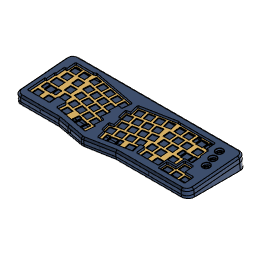
Trifecta (Autodesk Fusion 360 design; units mm, degrees)
Autodesk Fusion 360 part; units mm, degrees
(part 1 of 4)
sketch "plate" plane through (0, 0, 0) normal (0, 0, 1) x (1, 0, 0)
  arc A0 (312.6199, 117.774) -> (314.8699, 115.524) centre (314.8699, 117.774) ccw
  arc A1 (43.5915, -1.55) -> (40.3415, 1.7) centre (43.5915, 1.7) cw
  arc A2 (36.6259, 37.3436) -> (37.6259, 38.3436) centre (36.6259, 38.3436) ccw
  line L0 (175.886, -4.2231) -> (175.7904, -3.6814)
  arc A3 (112.7826, -2.4653) -> (110.9577, 0.1414) centre (110.5668, -2.0744) ccw
  arc A4 (31.0509, 50.8429) -> (30.0509, 49.8429) centre (31.0509, 49.8429) ccw
  arc A5 (179.6512, -6.859) -> (175.886, -4.2231) centre (179.0866, -3.6585) cw
  arc A6 (86.8114, 4.4012) -> (85.6822, 4.5) centre (85.6822, -2) ccw
  line L1 (47.3415, 2.25) -> (47.3415, 1.7)
  line L2 (-3.4991, 10) -> (-3.4991, 110.024)
  line L3 (312.6199, 118.324) -> (312.6199, 117.774)
  line L4 (26.1441, 107.024) -> (12.1447, 107.024)
  arc A7 (47.3415, 1.7) -> (44.0915, -1.55) centre (44.0915, 1.7) cw
  arc A8 (182.7796, -3.007) -> (180.1436, -6.7722) centre (179.579, -3.5716) cw
  line L5 (308.8699, 121.574) -> (309.3699, 121.574)
  line L6 (110.9577, 0.1414) -> (86.8114, 4.4012)
  line L7 (284.8904, 2.25) -> (284.8904, 1.7)
  line L8 (30.0509, 49.8429) -> (30.0509, 38.3436)
  arc A9 (115.323, -6.7722) -> (112.687, -3.007) centre (115.8876, -3.5716) cw
  line L9 (45.194, 107.024) -> (31.1947, 107.024)
  line L10 (112.687, -3.007) -> (112.7826, -2.4653)
  line L11 (352.994, 4.5) -> (287.1404, 4.5)
  circle A10 centre (133.6233, 118.074) radius 1.55
  arc A11 (277.8904, 2.25) -> (275.6404, 4.5) centre (275.6404, 2.25) ccw
  line L12 (12.0004, 37.3436) -> (6.4253, 37.3436)
  line L13 (40.3415, 1.7) -> (40.3415, 2.25)
  line L14 (305.6199, 117.774) -> (305.6199, 118.324)
  arc A12 (358.494, 10) -> (352.994, 4.5) centre (352.994, 10) cw
  line L15 (12.1447, 93.0243) -> (26.1441, 93.0243)
  line L16 (259.795, 93.0243) -> (273.794, 93.0243)
  line L17 (36.6259, 50.8429) -> (31.0509, 50.8429)
  line L18 (173.1838, -1.8565) -> (149.035, -6.1164)
  line L19 (146.4291, -6.1164) -> (122.2828, -1.8566)
  line L20 (180.1436, -6.7722) -> (179.6512, -6.859)
  line L21 (240.745, 107.024) -> (240.745, 93.0243)
  line L22 (208.6577, 4.4012) -> (184.5089, 0.1413)
  arc A13 (122.2828, -1.8566) -> (119.6762, -3.6815) centre (121.8919, -4.0724) ccw
  arc A14 (184.5089, 0.1413) -> (182.684, -2.4654) centre (184.8998, -2.0745) ccw
  arc A15 (40.3415, 2.25) -> (38.0915, 4.5) centre (38.0915, 2.25) ccw
  arc A16 (49.5915, 4.5) -> (47.3415, 2.25) centre (49.5915, 2.25) ccw
  line L23 (38.0915, 4.5) -> (2.0009, 4.5)
  arc A17 (13.0004, 38.3436) -> (12.0004, 37.3436) centre (12.0004, 38.3436) cw
  line L24 (115.8154, -6.859) -> (115.323, -6.7722)
  line L25 (288.37, 93.0243) -> (288.37, 107.024)
  arc A18 (309.3699, 121.574) -> (312.6199, 118.324) centre (309.3699, 118.324) cw
  line L26 (119.6762, -3.6815) -> (119.5806, -4.2231)
  line L27 (277.8904, 1.7) -> (277.8904, 2.25)
  arc A19 (303.3699, 115.524) -> (305.6199, 117.774) centre (303.3699, 117.774) ccw
  line L28 (358.494, 110.024) -> (358.494, 10)
  line L29 (31.0509, 37.3436) -> (36.6259, 37.3436)
  line L30 (13.0004, 49.8429) -> (13.0004, 38.3436)
  line L31 (182.684, -2.4654) -> (182.7796, -3.007)
  line L32 (85.6822, 4.5) -> (49.5915, 4.5)
  line L33 (174.9478, 20.2574) -> (176.9451, 8.9317)
  line L34 (303.895, 106.9941) -> (303.895, 95.4943)
  line L35 (98.9566, 12.3811) -> (100.9548, 23.7064)
  line L36 (314.754, 69.8941) -> (309.18, 69.8941)
  line L37 (283.556, 57.3947) -> (283.556, 68.8941)
  arc A20 (106.4177, 11.0651) -> (105.2592, 10.254) centre (105.4329, 11.2388) cw
  arc A21 (284.8904, 1.7) -> (281.6404, -1.55) centre (281.6404, 1.7) cw
  line L38 (304.895, 94.4943) -> (310.47, 94.4943)
  arc A22 (303.895, 95.4943) -> (304.895, 94.4943) centre (304.895, 95.4943) ccw
  line L39 (105.2592, 10.254) -> (99.7677, 11.2225)
  arc A23 (286.844, 95.4943) -> (285.844, 94.4943) centre (285.844, 95.4943) cw
  line L40 (279.269, 95.4943) -> (279.269, 106.9941)
  line L41 (315.754, 57.3947) -> (315.754, 68.8941)
  line L42 (130.6683, 6.7899) -> (132.6638, 18.1157)
  arc A24 (2.0009, 4.5) -> (-3.4991, 10) centre (2.0009, 10) cw
  arc A25 (287.1404, 4.5) -> (284.8904, 2.25) centre (287.1404, 2.25) ccw
  arc A26 (5.4253, 49.8429) -> (6.4253, 50.8429) centre (6.4253, 49.8429) cw
  line L43 (286.844, 106.9941) -> (286.844, 95.4943)
  arc A27 (314.754, 56.3947) -> (315.754, 57.3947) centre (314.754, 57.3947) ccw
  arc A28 (285.844, 107.9941) -> (286.844, 106.9941) centre (285.844, 106.9941) cw
  arc A29 (209.7869, 4.5) -> (208.6577, 4.4012) centre (209.7869, -2) ccw
  arc A30 (309.18, 69.8941) -> (308.18, 68.8941) centre (309.18, 68.8941) ccw
  line L44 (37.6259, 38.3436) -> (37.6259, 49.8429)
  arc A31 (305.6199, 118.324) -> (308.8699, 121.574) centre (308.8699, 118.324) cw
  arc A32 (126.3618, 20.2415) -> (125.2035, 19.4302) centre (126.1883, 19.2566) ccw
  arc A33 (191.7396, 23.2186) -> (192.5507, 24.3771) centre (192.7244, 23.3923) cw
  line L45 (281.6404, -1.55) -> (281.1404, -1.55)
  arc A34 (290.13, 69.8941) -> (291.13, 68.8941) centre (290.13, 68.8941) cw
  arc A35 (281.1404, -1.55) -> (277.8904, 1.7) centre (281.1404, 1.7) cw
  line L46 (227.1216, 115.524) -> (303.3699, 115.524)
  line L47 (124.0183, 6.9465) -> (129.5099, 5.9786)
  line L48 (131.8525, 19.274) -> (126.3618, 20.2415)
  line L49 (44.0915, -1.55) -> (43.5915, -1.55)
  arc A36 (30.0509, 38.3436) -> (31.0509, 37.3436) centre (31.0509, 38.3436) ccw
  line L50 (291.13, 68.8941) -> (291.13, 57.3947)
  arc A37 (310.47, 94.4943) -> (311.47, 95.4943) centre (310.47, 95.4943) ccw
  line L51 (309.18, 56.3947) -> (314.754, 56.3947)
  arc A38 (149.035, -6.1164) -> (146.4291, -6.1164) centre (147.7321, 1.2696) cw
  line L52 (275.6404, 4.5) -> (209.7869, 4.5)
  line L53 (125.2035, 19.4302) -> (123.207, 8.1049)
  line L54 (192.5507, 24.3771) -> (198.0375, 25.3445)
  arc A39 (119.5806, -4.2231) -> (115.8154, -6.859) centre (116.38, -3.6585) cw
  arc A40 (107.6038, 23.5487) -> (108.4148, 22.3903) centre (107.43, 22.564) cw
  line L55 (314.8699, 115.524) -> (352.994, 115.524)
  arc A41 (170.6459, 6.8059) -> (169.4875, 7.6172) centre (170.4724, 7.7907) cw
  arc A42 (167.4915, 18.9424) -> (168.3027, 20.1008) centre (168.4764, 19.116) cw
  arc A43 (99.7677, 11.2225) -> (98.9566, 12.3811) centre (99.9414, 12.2073) cw
  arc A44 (6.4253, 37.3436) -> (5.4253, 38.3436) centre (6.4253, 38.3436) cw
  arc A45 (291.13, 57.3947) -> (290.13, 56.3947) centre (290.13, 57.3947) cw
  line L56 (102.1133, 24.5174) -> (107.6038, 23.5487)
  arc A46 (175.7904, -3.6814) -> (173.1838, -1.8565) centre (173.5747, -4.0723) ccw
  arc A47 (352.994, 115.524) -> (358.494, 110.024) centre (352.994, 110.024) cw
  arc A48 (37.6259, 49.8429) -> (36.6259, 50.8429) centre (36.6259, 49.8429) ccw
  arc A49 (311.47, 106.9941) -> (310.47, 107.9941) centre (310.47, 106.9941) ccw
  line L57 (310.47, 107.9941) -> (304.895, 107.9941)
  line L58 (108.4148, 22.3903) -> (106.4177, 11.0651)
  line L59 (5.4253, 38.3436) -> (5.4253, 49.8429)
  arc A50 (129.5099, 5.9786) -> (130.6683, 6.7899) centre (129.6834, 6.9634) ccw
  arc A51 (100.9548, 23.7064) -> (102.1133, 24.5174) centre (101.9395, 23.5327) cw
  arc A52 (308.18, 57.3947) -> (309.18, 56.3947) centre (309.18, 57.3947) ccw
  line L60 (284.556, 69.8941) -> (290.13, 69.8941)
  line L61 (308.18, 68.8941) -> (308.18, 57.3947)
  line L62 (6.4253, 50.8429) -> (12.0004, 50.8429)
  arc A53 (315.754, 68.8941) -> (314.754, 69.8941) centre (314.754, 68.8941) ccw
  line L63 (290.13, 56.3947) -> (284.556, 56.3947)
  arc A54 (201.1942, 13.2086) -> (200.3832, 12.0501) centre (200.2094, 13.0348) cw
  arc A55 (173.7893, 21.0686) -> (174.9478, 20.2574) centre (173.963, 20.0838) cw
  line L64 (169.4875, 7.6172) -> (167.4915, 18.9424)
  arc A56 (123.207, 8.1049) -> (124.0183, 6.9465) centre (124.1918, 7.9313) ccw
  arc A57 (198.0375, 25.3445) -> (199.1959, 24.5335) centre (198.2111, 24.3597) cw
  line L65 (280.269, 107.9941) -> (285.844, 107.9941)
  arc A58 (304.895, 107.9941) -> (303.895, 106.9941) centre (304.895, 106.9941) ccw
  line L66 (200.3832, 12.0501) -> (194.8954, 11.0818)
  line L67 (285.844, 94.4943) -> (280.269, 94.4943)
  arc A59 (132.6638, 18.1157) -> (131.8525, 19.274) centre (131.679, 18.2892) ccw
  arc A60 (284.556, 56.3947) -> (283.556, 57.3947) centre (284.556, 57.3947) cw
  arc A61 (279.269, 106.9941) -> (280.269, 107.9941) centre (280.269, 106.9941) cw
  arc A62 (283.556, 68.8941) -> (284.556, 69.8941) centre (284.556, 68.8941) cw
  line L68 (168.3027, 20.1008) -> (173.7893, 21.0686)
  arc A63 (12.0004, 50.8429) -> (13.0004, 49.8429) centre (12.0004, 49.8429) cw
  line L69 (193.7369, 11.8929) -> (191.7396, 23.2186)
  arc A64 (176.9451, 8.9317) -> (176.1339, 7.7732) centre (175.9603, 8.758) cw
  arc A65 (280.269, 94.4943) -> (279.269, 95.4943) centre (280.269, 95.4943) cw
  arc A66 (194.8954, 11.0818) -> (193.7369, 11.8929) centre (194.7217, 12.0666) cw
  line L70 (311.47, 95.4943) -> (311.47, 106.9941)
  line L71 (176.1339, 7.7732) -> (170.6459, 6.8059)
  line L72 (199.1959, 24.5335) -> (201.1942, 13.2086)
  line L73 (209.276, 26.3412) -> (223.063, 28.7721)
  line L74 (307.132, 26.0615) -> (293.132, 26.0615)
  line L75 (117.549, 25.9388) -> (103.762, 28.3697)
  line L76 (101.221, 43.0332) -> (98.7887, 29.2475)
  line L77 (352.994, 115.024) -> (314.8699, 115.024)
  line L78 (215.434, 32.5548) -> (213.003, 46.3419)
  line L79 (229.222, 34.9856) -> (215.434, 32.5548)
  line L80 (307.132, 12.062) -> (307.132, 26.0615)
  line L81 (5.0009, 16.8245) -> (19.0004, 16.8245)
  line L82 (196.674, 29.2475) -> (194.243, 43.0332)
  line L83 (87.4339, 45.4642) -> (101.221, 43.0332)
  line L84 (312.182, 12.062) -> (326.182, 12.062)
  line L85 (293.132, 26.0615) -> (293.132, 12.062)
  line L86 (293.132, 12.062) -> (307.132, 12.062)
  line L87 (210.461, 31.6784) -> (196.674, 29.2475)
  line L88 (28.812, 16.8245) -> (42.8128, 16.8245)
  line L89 (226.791, 48.7729) -> (229.222, 34.9856)
  line L90 (66.2411, 34.9856) -> (68.6731, 48.7729)
  line L91 (106.193, 42.1569) -> (119.98, 39.726)
  line L92 (312.182, 45.1115) -> (312.182, 31.112)
  line L93 (124.955, 38.8482) -> (138.741, 36.4173)
  line L94 (326.182, 12.062) -> (326.182, 26.0615)
  line L95 (208.03, 45.4642) -> (210.461, 31.6784)
  line L96 (86.1882, 26.3412) -> (83.7558, 12.5525)
  arc A67 (357.994, 110.024) -> (352.994, 115.024) centre (352.994, 110.024) ccw
  line L97 (213.003, 46.3419) -> (226.791, 48.7729)
  line L98 (194.243, 43.0332) -> (208.03, 45.4642)
  line L99 (42.8128, 16.8245) -> (42.8128, 30.824)
  line L100 (309.3699, 121.074) -> (308.8699, 121.074)
  line L101 (19.0004, 16.8245) -> (19.0004, 30.824)
  line L102 (69.9685, 14.9848) -> (72.3995, 28.7721)
  line L103 (138.741, 36.4173) -> (136.31, 22.6315)
  line L104 (103.762, 28.3697) -> (106.193, 42.1569)
  line L105 (331.232, 26.0615) -> (331.232, 12.062)
  line L106 (223.063, 28.7721) -> (225.494, 14.9848)
  line L107 (156.722, 36.4173) -> (170.509, 38.8482)
  line L108 (72.3995, 28.7721) -> (86.1882, 26.3412)
  arc A68 (306.1199, 117.774) -> (303.3699, 115.024) centre (303.3699, 117.774) cw
  arc A69 (42.875, 117.774) -> (40.125, 115.024) centre (40.125, 117.774) cw
  line L109 (357.994, 10) -> (357.994, 110.024)
  line L110 (46.8415, 1.7) -> (46.8415, 2.25)
  line L111 (326.182, 45.1115) -> (312.182, 45.1115)
  line L112 (176.2828, -3.5946) -> (176.3784, -4.1362)
  line L113 (42.8128, 30.824) -> (28.812, 30.824)
  line L114 (306.1199, 118.324) -> (306.1199, 117.774)
  line L115 (184.4221, 0.6337) -> (208.5708, 4.8936)
  arc A70 (139.3733, 115.024) -> (136.6233, 117.774) centre (139.3733, 117.774) cw
  line L116 (82.459, 46.3419) -> (80.0283, 32.5548)
  line L117 (83.7558, 12.5525) -> (69.9685, 14.9848)
  line L118 (326.182, 26.0615) -> (312.182, 26.0615)
  line L119 (159.153, 22.6315) -> (156.722, 36.4173)
  line L120 (175.482, 39.726) -> (189.27, 42.1569)
  line L121 (19.0004, 30.824) -> (5.0009, 30.824)
  line L122 (345.232, 12.062) -> (345.232, 26.0615)
  line L123 (331.232, 12.062) -> (345.232, 12.062)
  line L124 (98.7887, 29.2475) -> (85.0015, 31.6784)
  line L125 (326.182, 31.112) -> (326.182, 45.1115)
  line L126 (218.3716, 118.324) -> (218.3716, 117.774)
  line L127 (136.31, 22.6315) -> (122.524, 25.0624)
  line L128 (136.6233, 117.774) -> (136.6233, 118.324)
  line L129 (68.6731, 48.7729) -> (82.459, 46.3419)
  line L130 (225.494, 14.9848) -> (211.708, 12.5525)
  line L131 (80.0283, 32.5548) -> (66.2411, 34.9856)
  line L132 (5.0009, 30.824) -> (5.0009, 16.8245)
  arc A71 (312.1199, 118.324) -> (309.3699, 121.074) centre (309.3699, 118.324) ccw
  line L133 (2.0009, 5) -> (38.0915, 5)
  line L134 (345.232, 26.0615) -> (331.232, 26.0615)
  line L135 (211.708, 12.5525) -> (209.276, 26.3412)
  line L136 (170.509, 38.8482) -> (172.94, 25.0624)
  line L137 (191.7, 28.3697) -> (177.913, 25.9388)
  arc A72 (314.8699, 115.024) -> (312.1199, 117.774) centre (314.8699, 117.774) cw
  line L138 (172.94, 25.0624) -> (159.153, 22.6315)
  line L139 (177.913, 25.9388) -> (175.482, 39.726)
  line L140 (189.27, 42.1569) -> (191.7, 28.3697)
  line L141 (312.182, 26.0615) -> (312.182, 12.062)
  line L142 (312.182, 31.112) -> (326.182, 31.112)
  line L143 (28.812, 30.824) -> (28.812, 16.8245)
  line L144 (85.0015, 31.6784) -> (87.4339, 45.4642)
  line L145 (113.275, -2.5522) -> (113.1794, -3.0938)
  line L146 (312.1199, 117.774) -> (312.1199, 118.324)
  line L147 (122.524, 25.0624) -> (124.955, 38.8482)
  line L148 (119.98, 39.726) -> (117.549, 25.9388)
  arc A73 (46.8415, 2.25) -> (49.5915, 5) centre (49.5915, 2.25) cw
  line L149 (42.875, 118.324) -> (42.875, 117.774)
  arc A74 (44.0915, -1.05) -> (46.8415, 1.7) centre (44.0915, 1.7) ccw
  arc A75 (2.0009, 115.024) -> (-2.9991, 110.024) centre (2.0009, 110.024) ccw
  arc A76 (218.3716, 117.774) -> (215.6216, 115.024) centre (215.6216, 117.774) cw
  line L150 (221.6216, 121.074) -> (221.1216, 121.074)
  arc A77 (308.8699, 121.074) -> (306.1199, 118.324) centre (308.8699, 118.324) ccw
  arc A78 (133.3733, 121.074) -> (130.6233, 118.324) centre (133.3733, 118.324) ccw
  arc A79 (119.1838, -3.5946) -> (122.3697, -1.3642) centre (121.8919, -4.0724) cw
  line L151 (115.4099, -6.2798) -> (115.9023, -6.3666)
  line L152 (224.3716, 117.774) -> (224.3716, 118.324)
  arc A80 (113.1794, -3.0938) -> (115.4099, -6.2798) centre (115.8876, -3.5716) ccw
  arc A81 (-2.9991, 10) -> (2.0009, 5) centre (2.0009, 10) ccw
  line L153 (49.5915, 5) -> (85.6822, 5)
  line L154 (119.0882, -4.1362) -> (119.1838, -3.5946)
  arc A82 (38.0915, 5) -> (40.8415, 2.25) centre (38.0915, 2.25) cw
  line L155 (303.3699, 115.024) -> (227.1216, 115.024)
  line L156 (48.875, 117.774) -> (48.875, 118.324)
  arc A83 (173.0969, -1.3641) -> (176.2828, -3.5946) centre (173.5747, -4.0723) cw
  line L157 (182.2872, -3.0939) -> (182.1916, -2.5522)
  line L158 (45.4822, 49.874) -> (45.4822, 35.8743)
  line L159 (195.341, 62.5711) -> (197.772, 48.7839)
  arc A84 (146.516, -5.624) -> (148.9482, -5.624) centre (147.7321, 1.2696) ccw
  line L160 (127.8733, 115.024) -> (51.625, 115.024)
  line L161 (122.3697, -1.3642) -> (146.516, -5.624)
  arc A85 (51.625, 115.024) -> (48.875, 117.774) centre (51.625, 117.774) cw
  arc A86 (85.6822, 5) -> (86.8983, 4.8935) centre (85.6822, -2) cw
  line L162 (133.8733, 121.074) -> (133.3733, 121.074)
  line L163 (281.1404, -1.05) -> (281.6404, -1.05)
  line L164 (349.994, 68.924) -> (335.995, 68.924)
  line L165 (281.226, 49.874) -> (281.226, 35.8743)
  arc A87 (208.5708, 4.8936) -> (209.7869, 5) centre (209.7869, -2) cw
  arc A88 (45.625, 121.074) -> (42.875, 118.324) centre (45.625, 118.324) ccw
  arc A89 (176.3784, -4.1362) -> (179.5643, -6.3666) centre (179.0866, -3.6585) ccw
  arc A90 (275.6404, 5) -> (278.3904, 2.25) centre (275.6404, 2.25) cw
  line L166 (215.6216, 115.024) -> (139.3733, 115.024)
  arc A91 (111.0446, 0.6338) -> (113.275, -2.5522) centre (110.5668, -2.0744) cw
  arc A92 (227.1216, 115.024) -> (224.3716, 117.774) centre (227.1216, 117.774) cw
  line L167 (40.125, 115.024) -> (2.0009, 115.024)
  line L168 (179.5643, -6.3666) -> (180.0567, -6.2798)
  line L169 (278.3904, 2.25) -> (278.3904, 1.7)
  arc A93 (48.875, 118.324) -> (46.125, 121.074) centre (46.125, 118.324) ccw
  line L170 (-2.9991, 110.024) -> (-2.9991, 10)
  line L171 (295.225, 35.8743) -> (295.225, 49.874)
  arc A94 (130.6233, 117.774) -> (127.8733, 115.024) centre (127.8733, 117.774) cw
  line L172 (235.982, 49.874) -> (235.982, 35.8743)
  line L173 (209.7869, 5) -> (275.6404, 5)
  arc A95 (352.994, 5) -> (357.994, 10) centre (352.994, 10) ccw
  arc A96 (221.1216, 121.074) -> (218.3716, 118.324) centre (221.1216, 118.324) ccw
  line L174 (116.451, 45.4752) -> (118.882, 59.2624)
  line L175 (46.125, 121.074) -> (45.625, 121.074)
  arc A97 (40.8415, 1.7) -> (43.5915, -1.05) centre (43.5915, 1.7) ccw
  line L176 (130.6233, 118.324) -> (130.6233, 117.774)
  arc A98 (136.6233, 118.324) -> (133.8733, 121.074) centre (133.8733, 118.324) ccw
  line L177 (249.982, 49.874) -> (235.982, 49.874)
  line L178 (86.8983, 4.8935) -> (111.0446, 0.6338)
  line L179 (45.4822, 35.8743) -> (59.4815, 35.8743)
  line L180 (14.5259, 49.874) -> (28.5254, 49.874)
  arc A99 (180.0567, -6.2798) -> (182.2872, -3.0939) centre (179.579, -3.5716) ccw
  line L181 (255.032, 49.874) -> (255.032, 35.8743)
  line L182 (28.5254, 35.8743) -> (14.5259, 35.8743)
  line L183 (43.5915, -1.05) -> (44.0915, -1.05)
  line L184 (165.224, 43.0445) -> (162.793, 56.8318)
  arc A100 (182.1916, -2.5522) -> (184.4221, 0.6337) centre (184.8998, -2.0745) cw
  line L185 (106.805, 13.2623) -> (106.8051, 13.2623)
  line L186 (269.032, 35.8743) -> (269.032, 49.874)
  line L187 (132.669, 56.8318) -> (130.238, 43.0445)
  line L188 (148.9482, -5.624) -> (173.0969, -1.3641)
  arc A101 (115.9023, -6.3666) -> (119.0882, -4.1362) centre (116.38, -3.6585) ccw
  arc A102 (224.3716, 118.324) -> (221.6216, 121.074) centre (221.6216, 118.324) ccw
  line L189 (197.772, 48.7839) -> (183.986, 46.3532)
  line L190 (176.444, 20.5521) -> (190.233, 22.9829)
  line L191 (235.982, 35.8743) -> (249.982, 35.8743)
  line L192 (335.995, 54.9243) -> (349.994, 54.9243)
  line L193 (281.226, 35.8743) -> (295.225, 35.8743)
  line L194 (249.982, 35.8743) -> (249.982, 49.874)
  line L195 (107.49, 8.3688) -> (109.921, 22.1561)
  line L196 (28.5254, 49.874) -> (28.5254, 35.8743)
  line L197 (40.8415, 2.25) -> (40.8415, 1.7)
  arc A103 (284.3904, 2.25) -> (287.1404, 5) centre (287.1404, 2.25) cw
  line L198 (280.938, 16.8245) -> (280.938, 30.824)
  line L199 (266.937, 30.824) -> (266.937, 16.8245)
  line L200 (81.3608, 65.8784) -> (95.148, 63.4478)
  line L201 (181.555, 60.1405) -> (195.341, 62.5711)
  line L202 (52.8147, 54.9243) -> (52.8147, 68.924)
  line L203 (111.478, 46.3532) -> (97.6905, 48.7839)
  line L204 (211.077, 84.6899) -> (224.864, 87.1209)
  line L205 (269.032, 73.9743) -> (269.032, 87.974)
  line L206 (306.655, 54.9243) -> (292.655, 54.9243)
  line L207 (59.4815, 35.8743) -> (59.4815, 49.874)
  line L208 (189.775, 66.7177) -> (175.988, 64.2867)
  line L209 (345.232, 87.974) -> (331.232, 87.974)
  line L210 (176.582, 59.2624) -> (179.013, 45.4752)
  line L211 (221.506, 52.9689) -> (219.075, 66.7561)
  line L212 (284.3904, 1.7) -> (284.3904, 2.25)
  line L213 (255.032, 35.8743) -> (269.032, 35.8743)
  line L214 (118.882, 59.2624) -> (132.669, 56.8318)
  line L215 (227.295, 73.3337) -> (213.509, 70.9027)
  line L216 (113.909, 60.1405) -> (111.478, 46.3532)
  line L217 (269.032, 87.974) -> (255.032, 87.974)
  line L218 (52.8147, 68.924) -> (38.8137, 68.924)
  line L219 (14.5259, 35.8743) -> (14.5259, 49.874)
  line L220 (257.125, 16.8245) -> (257.125, 30.824)
  arc A104 (281.6404, -1.05) -> (284.3904, 1.7) centre (281.6404, 1.7) ccw
  line L221 (269.032, 49.874) -> (255.032, 49.874)
  line L222 (109.921, 22.1561) -> (123.708, 19.7253)
  line L223 (178.876, 6.7634) -> (176.444, 20.5521)
  line L224 (280.938, 30.824) -> (266.937, 30.824)
  line L225 (121.277, 5.9366) -> (107.49, 8.3688)
  line L226 (130.238, 43.0445) -> (116.451, 45.4752)
  line L227 (266.937, 16.8245) -> (280.938, 16.8245)
  line L228 (162.793, 56.8318) -> (176.582, 59.2624)
  line L229 (107.6039, 17.7917) -> (107.603, 17.7919)
  line L230 (59.4815, 49.874) -> (45.4822, 49.874)
  line L231 (335.995, 68.924) -> (335.995, 54.9243)
  line L232 (192.664, 9.1957) -> (178.876, 6.7634)
  line L233 (168.785, 11.5852) -> (168.7882, 11.5858)
  line L234 (183.986, 46.3532) -> (181.555, 60.1405)
  line L235 (235.293, 55.3999) -> (221.506, 52.9689)
  line L236 (60.1694, 55.3999) -> (62.6001, 69.1871)
  line L237 (219.075, 66.7561) -> (232.862, 69.1871)
  line L238 (179.013, 45.4752) -> (165.224, 43.0445)
  line L239 (295.225, 49.874) -> (281.226, 49.874)
  line L240 (187.343, 80.5049) -> (189.775, 66.7177)
  line L241 (349.994, 54.9243) -> (349.994, 68.924)
  line L242 (345.232, 73.9743) -> (345.232, 87.974)
  line L243 (177.334, 6.7262) -> (177.334, 6.7262)
  line L244 (173.557, 78.0743) -> (187.343, 80.5049)
  line L245 (190.233, 22.9829) -> (192.664, 9.1956)
  line L246 (168.582, 77.1962) -> (171.013, 63.4104)
  line L247 (255.032, 73.9743) -> (269.032, 73.9743)
  line L248 (38.8137, 54.9243) -> (52.8147, 54.9243)
  line L249 (243.126, 30.824) -> (243.126, 16.8245)
  line L250 (257.125, 30.824) -> (243.126, 30.824)
  arc A105 (278.3904, 1.7) -> (281.1404, -1.05) centre (281.1404, 1.7) ccw
  line L251 (287.1404, 5) -> (352.994, 5)
  line L252 (123.708, 19.7253) -> (121.277, 5.9366)
  line L253 (95.148, 63.4478) -> (92.7171, 49.6605)
  line L254 (175.988, 64.2867) -> (173.557, 78.0743)
  line L255 (58.7872, 74.9886) -> (61.2179, 88.7748)
  line L256 (213.509, 70.9027) -> (211.077, 84.6899)
  line L257 (76.3873, 66.7561) -> (73.9567, 52.9689)
  line L258 (243.126, 16.8245) -> (257.125, 16.8245)
  line L259 (110.096, 65.9405) -> (96.3083, 68.3715)
  line L260 (275.7, 68.924) -> (261.699, 68.924)
  line L261 (171.013, 63.4104) -> (157.226, 60.9783)
  line L262 (75.0051, 86.3438) -> (72.5745, 72.5565)
  line L263 (292.655, 68.924) -> (306.655, 68.924)
  line L264 (249.982, 73.9743) -> (249.982, 87.974)
  line L265 (311.894, 87.974) -> (297.895, 87.974)
  line L266 (61.2179, 88.7748) -> (75.0051, 86.3438)
  line L267 (100.122, 62.5711) -> (113.909, 60.1405)
  line L268 (77.5476, 71.6802) -> (79.9786, 85.4675)
  line L269 (179.629, 98.4885) -> (193.416, 100.919)
  line L270 (182.059, 84.7012) -> (179.629, 98.4885)
  line L271 (193.416, 100.919) -> (195.847, 87.1319)
  line L272 (12.6201, 54.9243) -> (26.6209, 54.9243)
  line L273 (224.864, 87.1209) -> (227.295, 73.3337)
  line L274 (255.032, 87.974) -> (255.032, 73.9743)
  line L275 (202.747, 49.6605) -> (200.314, 63.4478)
  line L276 (214.103, 65.8784) -> (216.534, 52.0912)
  line L277 (130.189, 95.9584) -> (143.976, 93.5274)
  line L278 (174.655, 97.6119) -> (177.086, 83.8232)
  line L279 (256.65, 68.924) -> (242.649, 68.924)
  line L280 (297.895, 87.974) -> (297.895, 73.9743)
  line L281 (242.649, 54.9243) -> (256.65, 54.9243)
  line L282 (97.6905, 48.7839) -> (100.122, 62.5711)
  line L283 (12.1447, 73.9743) -> (26.1441, 73.9743)
  line L284 (73.9567, 52.9689) -> (60.1694, 55.3999)
  line L285 (112.527, 79.7278) -> (110.096, 65.9405)
  line L286 (331.232, 87.974) -> (331.232, 73.9743)
  line L287 (35.9572, 87.974) -> (35.9572, 73.9743)
  line L288 (275.7, 54.9243) -> (275.7, 68.924)
  line L289 (235.982, 87.974) -> (235.982, 73.9743)
  line L290 (261.699, 68.924) -> (261.699, 54.9243)
  line L291 (38.8137, 68.924) -> (38.8137, 54.9243)
  line L292 (230.937, 107.535) -> (233.368, 93.7479)
  line L293 (111.428, 99.2657) -> (125.214, 96.8347)
  line L294 (160.868, 95.1812) -> (174.655, 97.6119)
  line L295 (79.9786, 85.4675) -> (93.7659, 83.0365)
  line L296 (232.862, 69.1871) -> (235.293, 55.3999)
  line L297 (200.314, 63.4478) -> (214.103, 65.8784)
  line L298 (331.232, 73.9743) -> (345.232, 73.9743)
  line L299 (306.655, 68.924) -> (306.655, 54.9243)
  line L300 (35.9572, 73.9743) -> (49.9565, 73.9743)
  line L301 (274.082, 87.974) -> (274.082, 73.9743)
  line L302 (256.65, 54.9243) -> (256.65, 68.924)
  line L303 (292.655, 54.9243) -> (292.655, 68.924)
  line L304 (62.6001, 69.1871) -> (76.3873, 66.7561)
  line L305 (154.795, 74.7656) -> (168.582, 77.1962)
  line L306 (216.534, 52.0912) -> (202.747, 49.6605)
  line L307 (117.5, 78.8515) -> (131.287, 76.4205)
  line L308 (78.9298, 52.0912) -> (81.3608, 65.8784)
  line L309 (208.536, 70.0264) -> (194.747, 67.5954)
  line L310 (311.894, 73.9743) -> (311.894, 87.974)
  line L311 (96.3083, 68.3715) -> (98.7393, 82.1588)
  line L312 (261.699, 54.9243) -> (275.7, 54.9243)
  line L313 (115.069, 65.0642) -> (117.5, 78.8515)
  line L314 (98.7393, 82.1588) -> (112.527, 79.7278)
  line L315 (26.6209, 54.9243) -> (26.6209, 68.924)
  line L316 (26.6209, 68.924) -> (12.6201, 68.924)
  line L317 (72.5745, 72.5565) -> (58.7872, 74.9886)
  line L318 (92.7171, 49.6605) -> (78.9298, 52.0912)
  line L319 (297.895, 73.9743) -> (311.894, 73.9743)
  line L320 (242.649, 68.924) -> (242.649, 54.9243)
  line L321 (157.226, 60.9783) -> (154.795, 74.7656)
  line L322 (106.455, 100.143) -> (104.024, 86.3547)
  line L323 (104.024, 86.3547) -> (90.2353, 88.7857)
  line L324 (49.9565, 87.974) -> (35.9572, 87.974)
  line L325 (194.747, 67.5954) -> (192.316, 81.3816)
  line L326 (288.082, 73.9743) -> (288.082, 87.974)
  line L327 (177.086, 83.8232) -> (163.299, 81.3925)
  line L328 (90.2353, 88.7857) -> (92.6663, 102.574)
  line L329 (206.105, 83.8122) -> (208.536, 70.0264)
  line L330 (26.1441, 87.974) -> (12.1447, 87.974)
  line L331 (93.7659, 83.0365) -> (91.3349, 69.2492)
  line L332 (108.996, 85.4784) -> (111.428, 99.2657)
  line L333 (214.607, 90.4392) -> (200.82, 88.0085)
  line L334 (233.368, 93.7479) -> (219.581, 91.3172)
  line L335 (212.176, 104.228) -> (214.607, 90.4392)
  line L336 (143.976, 93.5274) -> (141.544, 79.7387)
  line L337 (92.6663, 102.574) -> (106.455, 100.143)
  line L338 (219.581, 91.3172) -> (217.15, 105.104)
  line L339 (26.1441, 73.9743) -> (26.1441, 87.974)
  line L340 (274.082, 73.9743) -> (288.082, 73.9743)
  line L341 (217.15, 105.104) -> (230.937, 107.535)
  line L342 (127.758, 82.1697) -> (130.189, 95.9584)
  line L343 (288.082, 87.974) -> (274.082, 87.974)
  line L344 (12.1447, 87.974) -> (12.1447, 73.9743)
  line L345 (195.847, 87.1319) -> (182.059, 84.7012)
  line L346 (200.82, 88.0085) -> (198.389, 101.797)
  line L347 (49.9565, 73.9743) -> (49.9565, 87.974)
  line L348 (122.783, 83.0474) -> (108.996, 85.4784)
  line L349 (128.856, 62.6332) -> (115.069, 65.0642)
  line L350 (249.982, 87.974) -> (235.982, 87.974)
  line L351 (163.299, 81.3925) -> (160.868, 95.1812)
  line L352 (141.544, 79.7387) -> (127.758, 82.1697)
  line L353 (198.389, 101.797) -> (212.176, 104.228)
  line L354 (192.316, 81.3816) -> (206.105, 83.8122)
  line L355 (131.287, 76.4205) -> (128.856, 62.6332)
  line L356 (235.982, 73.9743) -> (249.982, 73.9743)
  line L357 (125.214, 96.8347) -> (122.783, 83.0474)
  line L358 (87.6928, 103.451) -> (85.2622, 89.6634)
  line L359 (12.6201, 68.924) -> (12.6201, 54.9243)
  arc A106 (137.1233, 117.774) -> (139.3733, 115.524) centre (139.3733, 117.774) ccw
  arc A107 (217.8716, 118.324) -> (221.1216, 121.574) centre (221.1216, 118.324) cw
  line L360 (71.476, 92.0944) -> (73.9069, 105.882)
  line L361 (326.47, 107.024) -> (326.47, 93.0243)
  line L362 (51.625, 115.524) -> (127.8733, 115.524)
  line L363 (26.1441, 93.0243) -> (26.1441, 107.024)
  arc A108 (133.8733, 121.574) -> (137.1233, 118.324) centre (133.8733, 118.324) cw
  line L364 (45.194, 93.0243) -> (45.194, 107.024)
  line L365 (259.795, 107.024) -> (259.795, 93.0243)
  line L366 (254.744, 107.024) -> (240.745, 107.024)
  arc A109 (-3.4991, 110.024) -> (2.0009, 115.524) centre (2.0009, 110.024) cw
  circle A110 centre (309.1199, 118.074) radius 1.55
  line L367 (254.744, 93.0243) -> (254.744, 107.024)
  line L368 (52.7142, 95.4017) -> (55.1448, 109.19)
  line L369 (31.1947, 93.0243) -> (45.194, 93.0243)
  line L370 (340.469, 93.0243) -> (340.469, 107.024)
  line L371 (45.625, 121.574) -> (46.125, 121.574)
  line L372 (139.3733, 115.524) -> (215.6216, 115.524)
  line L373 (240.745, 93.0243) -> (254.744, 93.0243)
  line L374 (12.1447, 107.024) -> (12.1447, 93.0243)
  line L375 (73.9069, 105.882) -> (87.6928, 103.451)
  line L376 (273.794, 93.0243) -> (273.794, 107.024)
  arc A111 (221.6216, 121.574) -> (224.8716, 118.324) centre (221.6216, 118.324) cw
  circle A112 centre (179.2893, -3.3688) radius 1.55
  circle A113 centre (116.1773, -3.3688) radius 1.55
  arc A114 (130.1233, 118.324) -> (133.3733, 121.574) centre (133.3733, 118.324) cw
  line L377 (91.3349, 69.2492) -> (77.5476, 71.6802)
  circle A115 centre (43.8415, 1.95) radius 1.55
  line L378 (49.375, 118.324) -> (49.375, 117.774)
  arc A116 (224.8716, 117.774) -> (227.1216, 115.524) centre (227.1216, 117.774) ccw
  line L379 (224.8716, 118.324) -> (224.8716, 117.774)
  line L380 (85.2622, 89.6634) -> (71.476, 92.0944)
  line L381 (137.1233, 118.324) -> (137.1233, 117.774)
  line L382 (55.1448, 109.19) -> (68.9335, 106.759)
  circle A117 centre (45.875, 118.074) radius 1.55
  circle A118 centre (281.3904, 1.95) radius 1.55
  line L383 (66.5014, 92.9707) -> (52.7142, 95.4017)
  line L384 (31.1947, 107.024) -> (31.1947, 93.0243)
  circle A119 centre (221.3716, 118.074) radius 1.55
  line L385 (288.37, 107.024) -> (302.369, 107.024)
  arc A120 (40.125, 115.524) -> (42.375, 117.774) centre (40.125, 117.774) ccw
  line L386 (2.0009, 115.524) -> (40.125, 115.524)
  line L387 (68.9335, 106.759) -> (66.5014, 92.9707)
  arc A121 (215.6216, 115.524) -> (217.8716, 117.774) centre (215.6216, 117.774) ccw
  arc A122 (46.125, 121.574) -> (49.375, 118.324) centre (46.125, 118.324) cw
  line L388 (326.47, 93.0243) -> (340.469, 93.0243)
  arc A123 (42.375, 118.324) -> (45.625, 121.574) centre (45.625, 118.324) cw
  arc A124 (127.8733, 115.524) -> (130.1233, 117.774) centre (127.8733, 117.774) ccw
  line L389 (133.3733, 121.574) -> (133.8733, 121.574)
  arc A125 (49.375, 117.774) -> (51.625, 115.524) centre (51.625, 117.774) ccw
  line L390 (221.1216, 121.574) -> (221.6216, 121.574)
  line L391 (273.794, 107.024) -> (259.795, 107.024)
  line L392 (217.8716, 117.774) -> (217.8716, 118.324)
  line L393 (130.1233, 117.774) -> (130.1233, 118.324)
  line L394 (340.469, 107.024) -> (326.47, 107.024)
  line L395 (302.369, 93.0243) -> (288.37, 93.0243)
  line L396 (302.369, 107.024) -> (302.369, 93.0243)
  line L397 (42.375, 117.774) -> (42.375, 118.324)
  line L398 (7.8576, 68.924) -> (7.8576, 54.9243)
  line L399 (7.8576, 68.924) -> (12.6201, 68.924)
  line L400 (7.8576, 54.9243) -> (12.6201, 54.9243)
  line L401 (359.744, 110.024) -> (359.744, 10)
  arc A126 (352.994, 3.25) -> (359.744, 10) centre (352.994, 10) ccw
  line L402 (352.994, 3.25) -> (287.1404, 3.25)
  arc A127 (287.1404, 3.25) -> (286.1404, 2.25) centre (287.1404, 2.25) ccw
  line L403 (286.1404, 2.25) -> (286.1404, 1.7)
  arc A128 (281.6404, -2.8) -> (286.1404, 1.7) centre (281.6404, 1.7) ccw
  line L404 (281.6404, -2.8) -> (281.1404, -2.8)
  arc A129 (276.6404, 1.7) -> (281.1404, -2.8) centre (281.1404, 1.7) ccw
  line L405 (276.6404, 1.7) -> (276.6404, 2.25)
  arc A130 (276.6404, 2.25) -> (275.6404, 3.25) centre (275.6404, 2.25) ccw
  line L406 (275.6404, 3.25) -> (209.7869, 3.25)
  arc A131 (209.7869, 3.25) -> (208.8748, 3.1702) centre (209.7869, -2) ccw
  line L407 (208.8748, 3.1702) -> (184.7261, -1.0897)
  arc A132 (184.7261, -1.0897) -> (183.915, -2.2482) centre (184.8998, -2.0745) ccw
  line L408 (183.915, -2.2482) -> (184.0105, -2.7899)
  arc A133 (180.3607, -8.0032) -> (184.0105, -2.7899) centre (179.579, -3.5716) ccw
  line L409 (180.3607, -8.0032) -> (179.8683, -8.09)
  arc A134 (174.655, -4.4402) -> (179.8683, -8.09) centre (179.0866, -3.6585) ccw
  line L410 (174.655, -4.4402) -> (174.5594, -3.8986)
  arc A135 (174.5594, -3.8986) -> (173.4009, -3.0875) centre (173.5747, -4.0723) ccw
  line L411 (173.4009, -3.0875) -> (149.2522, -7.3474)
  arc A136 (146.212, -7.3474) -> (149.2522, -7.3474) centre (147.7321, 1.2696) ccw
  line L412 (146.212, -7.3474) -> (122.0657, -3.0876)
  arc A137 (122.0657, -3.0876) -> (120.9071, -3.8986) centre (121.8919, -4.0724) ccw
  line L413 (120.9071, -3.8986) -> (120.8116, -4.4403)
  arc A138 (115.5982, -8.09) -> (120.8116, -4.4403) centre (116.38, -3.6585) ccw
  line L414 (115.5982, -8.09) -> (115.1058, -8.0032)
  arc A139 (111.4561, -2.7898) -> (115.1058, -8.0032) centre (115.8876, -3.5716) ccw
  line L415 (111.4561, -2.7898) -> (111.5516, -2.2482)
  arc A140 (111.5516, -2.2482) -> (110.7406, -1.0896) centre (110.5668, -2.0744) ccw
  line L416 (110.7406, -1.0896) -> (86.5943, 3.1702)
  arc A141 (86.5943, 3.1702) -> (85.6822, 3.25) centre (85.6822, -2) ccw
  line L417 (85.6822, 3.25) -> (49.5915, 3.25)
  arc A142 (49.5915, 3.25) -> (48.5915, 2.25) centre (49.5915, 2.25) ccw
  line L418 (48.5915, 2.25) -> (48.5915, 1.7)
  arc A143 (44.0915, -2.8) -> (48.5915, 1.7) centre (44.0915, 1.7) ccw
  line L419 (44.0915, -2.8) -> (43.5915, -2.8)
  arc A144 (39.0915, 1.7) -> (43.5915, -2.8) centre (43.5915, 1.7) ccw
  line L420 (39.0915, 1.7) -> (39.0915, 2.25)
  arc A145 (39.0915, 2.25) -> (38.0915, 3.25) centre (38.0915, 2.25) ccw
  line L421 (38.0915, 3.25) -> (2.0009, 3.25)
  arc A146 (-4.7491, 10) -> (2.0009, 3.25) centre (2.0009, 10) ccw
  line L422 (-4.7491, 10) -> (-4.7491, 110.024)
  arc A147 (2.0009, 116.774) -> (-4.7491, 110.024) centre (2.0009, 110.024) ccw
  line L423 (2.0009, 116.774) -> (40.125, 116.774)
  arc A148 (40.125, 116.774) -> (41.125, 117.774) centre (40.125, 117.774) ccw
  line L424 (41.125, 117.774) -> (41.125, 118.324)
  arc A149 (45.625, 122.824) -> (41.125, 118.324) centre (45.625, 118.324) ccw
  line L425 (45.625, 122.824) -> (46.125, 122.824)
  arc A150 (50.625, 118.324) -> (46.125, 122.824) centre (46.125, 118.324) ccw
  line L426 (50.625, 118.324) -> (50.625, 117.774)
  arc A151 (50.625, 117.774) -> (51.625, 116.774) centre (51.625, 117.774) ccw
  line L427 (51.625, 116.774) -> (127.8733, 116.774)
  arc A152 (127.8733, 116.774) -> (128.8733, 117.774) centre (127.8733, 117.774) ccw
  line L428 (128.8733, 117.774) -> (128.8733, 118.324)
  arc A153 (133.3733, 122.824) -> (128.8733, 118.324) centre (133.3733, 118.324) ccw
  line L429 (133.3733, 122.824) -> (133.8733, 122.824)
  arc A154 (138.3733, 118.324) -> (133.8733, 122.824) centre (133.8733, 118.324) ccw
  line L430 (138.3733, 118.324) -> (138.3733, 117.774)
  arc A155 (138.3733, 117.774) -> (139.3733, 116.774) centre (139.3733, 117.774) ccw
  line L431 (139.3733, 116.774) -> (215.6216, 116.774)
  arc A156 (215.6216, 116.774) -> (216.6216, 117.774) centre (215.6216, 117.774) ccw
  line L432 (216.6216, 117.774) -> (216.6216, 118.324)
  arc A157 (221.1216, 122.824) -> (216.6216, 118.324) centre (221.1216, 118.324) ccw
  line L433 (221.1216, 122.824) -> (221.6216, 122.824)
  arc A158 (226.1216, 118.324) -> (221.6216, 122.824) centre (221.6216, 118.324) ccw
  line L434 (226.1216, 118.324) -> (226.1216, 117.774)
  arc A159 (226.1216, 117.774) -> (227.1216, 116.774) centre (227.1216, 117.774) ccw
  line L435 (227.1216, 116.774) -> (303.3699, 116.774)
  arc A160 (303.3699, 116.774) -> (304.3699, 117.774) centre (303.3699, 117.774) ccw
  line L436 (304.3699, 117.774) -> (304.3699, 118.324)
  arc A161 (308.8699, 122.824) -> (304.3699, 118.324) centre (308.8699, 118.324) ccw
  line L437 (308.8699, 122.824) -> (309.3699, 122.824)
  arc A162 (313.8699, 118.324) -> (309.3699, 122.824) centre (309.3699, 118.324) ccw
  line L438 (313.8699, 118.324) -> (313.8699, 117.774)
  arc A163 (313.8699, 117.774) -> (314.8699, 116.774) centre (314.8699, 117.774) ccw
  line L439 (314.8699, 116.774) -> (352.994, 116.774)
  arc A164 (359.744, 110.024) -> (352.994, 116.774) centre (352.994, 110.024) ccw
  dimension "d54" = -1.25
  constraint perpendicular L359 L399
  constraint perpendicular L359 L400
extrude "plate (1)" add sketch "plate" along normal blind 1.6 contours A0 A1 L0 A3 A5 A6 L1 L2 L3 A7 A8 L5 L6 L7 A9 L10 L11 A11 L13 L14 A12 L18 L19 L20 L22 A13 A14 A15 A16 L23 L24 A18 L26 L27 A19 L28 L31 L32 A21 A24 A25 A29 A31 L45 A35 L46 L49 A38 L52 A39 L55 A46 A47 A106 A107 L362 A108 A109 L371 L372 A111 A114 L378 A116 L379 L381 A120 L386 A121 A122 A123 A124 L389 A125 L390 L392 L393 L397 | L77 A67 L100 A68 A69 L109 L110 L112 L114 L115 A70 L126 L128 A71 L133 A72 L145 L146 A73 L149 A74 A75 A76 L150 A77 A78 A79 L151 L152 A80 A81 L153 L154 A82 L155 L156 A83 L157 A84 L160 L161 A85 A86 L162 L163 A87 A88 A89 A90 L166 A91 A92 L167 L168 L169 A93 L170 A94 L173 A95 A96 L175 A97 L176 A98 L178 A99 L183 A100 L188 A101 A102 L197 A103 L212 A104 A105 L251 makes body 1